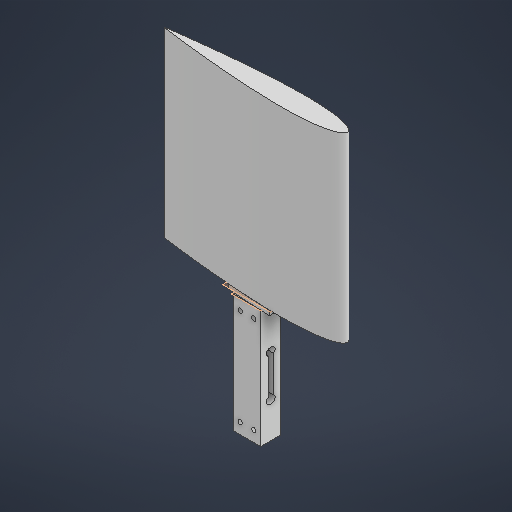
# Autodesk Inventor part: Suporte
Saved by Autodesk Inventor 2027.1 (Build 311270010, 270A)
## iProperties
Created: 2026-08-03
Part Number: Suporte
Material: Genérico
Document SubType Name: Modeling
Designer: mateu
Density: 1 g/cm^3
Appearance: Padrão
Author: mateu
Autodesk Inventor part; units mm, degrees
ref_plane "YZ Plane" through (0, 0, 0) normal (1, 0, 0) x (0, 1, 0)
ref_plane "XZ Plane" through (0, 0, 0) normal (0, 1, 0) x (-1, 0, 0)
ref_plane "XY Plane" through (0, 0, 0) normal (0, 0, 1) x (1, 0, 0)
sketch "Esboço1" plane through (0, 0, 0) normal (0, 0, 1) x (1, 0, 0)
  line L0 (-15, 65) -> (15, 65)
  line L1 (15, 65) -> (15, -65)
  line L2 (15, -65) -> (-15, -65)
  line L3 (-15, -65) -> (-15, 65)
  point P0 (0, 0)
  point P1 (0, 65)
  dimension "d0" = 130
  dimension "d1" = 65
  dimension "d2" = 30
  dimension "d3" = 0
  constraints: 8 end point, 2 parallel, 1 horizontal, 1 midpoint, 1 perpendicular
  measures "d0" distance of L1.end L0.end
  measures "d1" distance from line of point (0, 0) L0
  measures "d2" distance of L0.end L0.start
  measures "d3" horizontal distance of point (0, 65) point (0, 0)
extrude "Extrusão1" add sketch "Esboço1" along normal blind 22
sketch "Esboço2" plane through (0, 0, 0) normal (0, 0, -1) x (-1, 0, 0)
  line L0 (15, -65) -> (-15, -65) projected
  line L1 (15, 65) -> (15, -65) projected
  point P0 (0, 0)
  point P1 (7.5, -53)
  point P2 (0, -65)
  dimension "d24" = 7.5
  dimension "d25" = 12
  constraints: 1 midpoint
  measures "d24" distance from line of L1 point (7.5, -53)
  measures "d25" distance from line of L0 point (7.5, -53)
hole "Furo1" at (-7.5, -53, 0) direction (0, 0, 1) diameter 4.917 end through all thread size "M6x1" class "6H" standard "ISO Metric profile"
sketch "Esboço3" plane through (0, 0, 0) normal (0, 0, -1) x (-1, 0, 0)
  line L0 (15, -65) -> (-15, -65) projected
  circle A0 centre (7.5, -53) radius 2.4585 projected
  point P0 (0, 0)
  point P1 (-7.5, -53)
  dimension "d22" = 12
  dimension "d26" = 15
  measures "d22" distance from line of L0 point (-7.5, -53)
  measures "d26" distance of point (-7.5, -53) A0.centre
hole "Furo2" at (7.5, -53, 0) direction (0, 0, 1) diameter 4.917 end through all thread size "M6x1" class "6H" standard "ISO Metric profile"
sketch "Esboço4" plane through (0, 0, 22) normal (0, 0, 1) x (1, 0, 0)
  line L0 (15, 65) -> (-15, 65) projected
  line L1 (15, -65) -> (15, 65) projected
  point P0 (0, 0)
  point P1 (-7.5, 53)
  point P2 (7.5, 53)
  dimension "d34" = 15
  dimension "d35" = 12
  dimension "d36" = 12
  dimension "d37" = 7.5
  measures "d34" distance of point (7.5, 53) point (-7.5, 53)
  measures "d35" distance from line of L0 point (-7.5, 53)
  measures "d36" distance from line of L0 point (7.5, 53)
  measures "d37" distance from line of L1 point (7.5, 53)
hole "Furo3" at (-7.5, 53, 22) at (7.5, 53, 22) direction (0, 0, -1) diameter 4.917 end through all thread size "M6x1" class "6H" standard "ISO Metric profile"
sketch "Esboço5" plane through (-15, -65, 0) normal (-1, 0, 0) x (0, 0, 1)
  line L0 (8, 42.2) -> (8, 81.8)
  line L1 (22, 0) -> (22, 130) projected
  line L2 (13.2941, 42.5541) -> (13.2941, 81.4459)
  line L3 (0, 130) -> (0, 0) projected
  ellipse E0 centre (11, 39) end of major axis (6, 39) minor radius 4 (8, 42.2) -> (13.2941, 42.5541) ccw
  ellipse E1 centre (11, 85) end of major axis (6, 85) minor radius 4 (13.2941, 81.4459) -> (8, 81.8) ccw
  point P0 (0, 65)
  point P1 (0, 65)
  point P2 (8, 62)
  dimension "d40" = 8
  constraints: 4 end point, 2 midpoint, 1 vertical, 8 other
  measures "d40" horizontal distance of point (0, 65) point (8, 62)
extrude "Extrusão2" cut sketch "Esboço5" against normal blind 30
sketch "Esboço6" plane through (-15, 65, 0) normal (0, 1, 0) x (1, 0, 0)
  line L0 (30, 0) -> (0, 0) projected
  line L1 (30, 0) -> (30, -22) projected
  point P0 (15, 0)
  point P1 (15, -11)
  point P2 (15, 0)
  dimension "d50" = 11
  dimension "d51" = 15
  constraints: 1 midpoint
  measures "d50" distance of point (15, 0) point (15, -11)
  measures "d51" distance from line of L1 point (15, -11)
hole "Furo4" at (0, 65, 11) direction (0, -1, 0) diameter 4.917 end through all thread size "M6x1" class "6H" standard "ISO Metric profile"
ref_plane "Plano de trabalho1" through (-15, 65, 11) normal (0, 1, 0) x (1, 0, 0)
sketch "Esboço7" plane through (-15, 65, 0) normal (0, 1, 0) x (1, 0, 0)
  spline S0 degree 4 poles (-85.9155, -11.2779) (-85.8439, -11.2878) (-85.4953, -11.3359) (-84.9101, -11.4167) (-83.9238, -11.5521) (-82.8882, -11.6927) (-81.6192, -11.8648) (-80.129, -12.0648) (-78.4169, -12.2921) (-76.4894, -12.5454) (-74.3498, -12.823) (-72.0038, -13.1236) (-69.4563, -13.4446) (-66.7141, -13.7854) (-63.7826, -14.1434) (-60.6694, -14.5168) (-57.3818, -14.904) (-53.9268, -15.3029) (-50.3132, -15.7109) (-46.549, -16.1274) (-42.6432, -16.5489) (-38.605, -16.9747) (-34.4437, -17.4012) (-30.1687, -17.8282) (-25.7912, -18.2519) (-21.3189, -18.671) (-16.7725, -19.0832) (-12.1287, -19.4848) (-7.4947, -19.8798) (-2.7032, -20.2527) (2.0551, -20.6151) (6.8684, -20.956) (11.6887, -21.2762) (16.5168, -21.572) (21.3384, -21.8407) (26.1391, -22.0803) (30.9224, -22.2877) (35.6373, -22.462) (40.3236, -22.599) (44.9725, -22.6969) (49.5196, -22.7548) (53.9946, -22.7699) (58.3721, -22.741) (62.6467, -22.6675) (66.8074, -22.5469) (70.8451, -22.3803) (74.7504, -22.1661) (78.514, -21.9053) (82.1273, -21.5976) (85.5816, -21.2439) (88.8692, -20.8453) (91.9823, -20.4037) (94.9136, -19.9196) (97.6566, -19.3956) (100.2049, -18.8338) (102.5526, -18.2359) (104.6947, -17.6047) (106.6265, -16.9423) (108.3443, -16.2508) (109.8449, -15.5323) (111.1261, -14.7877) (112.1867, -14.0178) (113.0249, -13.2201) (113.6369, -12.3914) (114.0114, -11.531) (114.1354, -10.6418) (114.008, -9.7531) (113.6302, -8.8941) (113.015, -8.0678) (112.1737, -7.2733) (111.1102, -6.5075) (109.8262, -5.7678) (108.3229, -5.0551) (106.6024, -4.3702) (104.6681, -3.7152) (102.5235, -3.0923) (100.1736, -2.5034) (97.6231, -1.9513) (94.8781, -1.4379) (91.945, -0.965) (88.8302, -0.5354) (85.5411, -0.1494) (82.0855, 0.1911) (78.471, 0.4848) (74.7065, 0.7312) (70.8004, 0.9304) (66.7621, 1.0815) (62.6007, 1.1861) (58.3266, 1.2432) (53.9484, 1.2553) (49.4819, 1.223) (44.9219, 1.1481) (40.3202, 1.0315) (35.6328, 0.8761) (30.8735, 0.6853) (26.1044, 0.4588) (21.296, 0.2008) (16.4759, -0.0866) (11.6491, -0.4009) (6.8288, -0.7393) (2.0251, -1.0991) (-2.7506, -1.4782) (-7.4865, -1.8734) (-12.1725, -2.2823) (-16.7969, -2.7033) (-21.3494, -3.1325) (-25.8188, -3.5691) (-30.1955, -4.0095) (-34.4685, -4.453) (-38.6282, -4.8954) (-42.6647, -5.3367) (-46.5689, -5.7732) (-50.3314, -6.2041) (-53.9435, -6.626) (-57.3969, -7.0382) (-60.683, -7.438) (-63.7948, -7.8234) (-66.7248, -8.1926) (-69.4657, -8.544) (-72.0119, -8.8747) (-74.3568, -9.1844) (-76.4953, -9.4701) (-78.4218, -9.7309) (-80.133, -9.9648) (-81.6225, -10.1704) (-82.8907, -10.3474) (-83.9258, -10.492) (-84.9116, -10.6312) (-85.4965, -10.7142) (-85.8449, -10.7636) (-85.9164, -10.7739) knots 0 0 0 0 0 0.0063 0.010007 0.01432 0.019151 0.024442 0.030148 0.036235 0.042672 0.049434 0.056497 0.063841 0.071448 0.079299 0.087378 0.09567 0.104159 0.112831 0.121672 0.130669 0.139808 0.149077 0.158464 0.167955 0.177539 0.187194 0.196927 0.206717 0.216551 0.226428 0.236317 0.246216 0.256114 0.265998 0.275852 0.28567 0.295446 0.305162 0.314814 0.324383 0.333852 0.343216 0.352462 0.361579 0.370555 0.379378 0.388035 0.396515 0.404804 0.412889 0.420757 0.428395 0.435788 0.442923 0.449784 0.456357 0.462627 0.468581 0.47421 0.479508 0.484483 0.489162 0.493602 0.497886 0.502114 0.506398 0.510839 0.515517 0.520492 0.52579 0.531419 0.537373 0.543644 0.550217 0.557078 0.564212 0.571605 0.579243 0.587112 0.595197 0.603486 0.611965 0.620622 0.629445 0.638421 0.647538 0.656784 0.666148 0.675617 0.685175 0.694814 0.704531 0.714306 0.724136 0.734001 0.743886 0.753783 0.763683 0.773572 0.78344 0.793274 0.803064 0.812797 0.822461 0.832045 0.841536 0.850923 0.860192 0.869331 0.878328 0.887169 0.895841 0.90433 0.912622 0.920701 0.928552 0.936159 0.943503 0.950566 0.957328 0.963765 0.969852 0.975558 0.980849 0.98568 0.989993 0.9937 1 1 1 1 1
  line L0 (-85.4498, -10.7076) -> (-85.9164, -10.7739)
  line L1 (-85.7986, -11.294) -> (-87.8652, -11.0296)
  line L2 (-87.8652, -11.0296) -> (-85.7997, -10.7572)
  arc A0 (-13.9447, 8.0586) -> (-13.9447, 8.0586) centre (-12.476, -36.7013) ccw
  line L3 (96.9543, 74.8341) -> (75.7631, 39.7352)
  circle A1 centre (85.6496, 3.5164) radius 2.75
  line L4 (85.6496, 3.5164) -> (84.9837, -0.1033)
  line L5 (30, -22) -> (0, -22) projected
  line L6 (40.3546, 1.025) -> (40.3546, -22.5918)
  line L7 (-7.5118, -1.8793) -> (-7.5118, -19.8713)
  circle A2 centre (15, -11) radius 2.4585
  point P0 (15, 0)
  point P1 (-12.476, -36.7013)
  point P2 (-85.4485, -11.3424)
  point P3 (-84.8658, -11.4227)
  point P4 (-84.052, -11.5343)
  point P5 (-83.0089, -11.6763)
  point P6 (-81.739, -11.8483)
  point P7 (-80.2452, -12.0488)
  point P8 (-78.5309, -12.2765)
  point P9 (-76.6004, -12.5302)
  point P10 (-74.4581, -12.8083)
  point P11 (-72.1089, -13.1092)
  point P12 (-69.5583, -13.4309)
  point P13 (-66.8124, -13.772)
  point P14 (-63.8773, -14.1306)
  point P15 (-60.7602, -14.5046)
  point P16 (-57.4685, -14.8923)
  point P17 (-54.0093, -15.2916)
  point P18 (-50.3911, -15.7005)
  point P19 (-46.6223, -16.1172)
  point P20 (-42.7117, -16.5395)
  point P21 (-38.6685, -16.9656)
  point P22 (-34.502, -17.393)
  point P23 (-30.222, -17.8202)
  point P24 (-25.8384, -18.2445)
  point P25 (-21.3618, -18.6641)
  point P26 (-16.8022, -19.0766)
  point P27 (-12.1704, -19.4799)
  point P28 (-2.7339, -20.2486)
  point P29 (2.049, -20.6094)
  point P30 (6.8599, -20.951)
  point P31 (11.6875, -21.2709)
  point P32 (16.5209, -21.5666)
  point P33 (21.3484, -21.8354)
  point P34 (26.1591, -22.0747)
  point P35 (30.9415, -22.2821)
  point P36 (35.6622, -22.4553)
  point P37 (45.0083, -22.6895)
  point P38 (49.5672, -22.7464)
  point P39 (54.0432, -22.7606)
  point P40 (58.426, -22.7308)
  point P41 (62.7051, -22.6558)
  point P42 (66.8704, -22.5342)
  point P43 (70.9125, -22.3658)
  point P44 (74.8219, -22.1501)
  point P45 (78.5894, -21.8873)
  point P46 (82.2062, -21.5775)
  point P47 (85.6637, -21.2215)
  point P48 (88.9542, -20.8204)
  point P49 (92.0697, -20.3756)
  point P50 (95.003, -19.8883)
  point P51 (97.7474, -19.3607)
  point P52 (100.2963, -18.7946)
  point P53 (102.6438, -18.1921)
  point P54 (104.7843, -17.5556)
  point P55 (106.7131, -16.8873)
  point P56 (108.4255, -16.1894)
  point P57 (109.9175, -15.4641)
  point P58 (111.1857, -14.7135)
  point P59 (112.227, -13.9397)
  point P60 (113.0391, -13.1441)
  point P61 (113.6201, -12.3286)
  point P62 (113.9685, -11.4941)
  point P63 (114.0837, -10.6419)
  point P64 (113.9653, -9.7901)
  point P65 (113.6137, -8.957)
  point P66 (113.0295, -8.1437)
  point P67 (112.2144, -7.3513)
  point P68 (111.1701, -6.5815)
  point P69 (109.8991, -5.8357)
  point P70 (108.4043, -5.1162)
  point P71 (106.6891, -4.4249)
  point P72 (104.7579, -3.764)
  point P73 (102.6149, -3.1357)
  point P74 (100.2651, -2.5422)
  point P75 (97.714, -1.9859)
  point P76 (94.9676, -1.4688)
  point P77 (92.0325, -0.9928)
  point P78 (88.9153, -0.56)
  point P79 (85.6233, -0.1715)
  point P80 (82.1645, 0.1712)
  point P81 (78.5465, 0.4671)
  point P82 (74.778, 0.7155)
  point P83 (70.8678, 0.9162)
  point P84 (66.8251, 1.069)
  point P85 (62.6593, 1.1746)
  point P86 (58.38, 1.2332)
  point P87 (53.9972, 1.2462)
  point P88 (49.5212, 1.2148)
  point P89 (44.9625, 1.1404)
  point P90 (35.6622, 0.8703)
  point P91 (30.8974, 0.679)
  point P92 (26.1158, 0.4532)
  point P93 (21.3061, 0.1954)
  point P94 (16.4797, -0.0919)
  point P95 (11.6474, -0.4061)
  point P96 (6.8211, -0.7446)
  point P97 (2.0116, -1.1046)
  point P98 (-2.7699, -1.4838)
  point P99 (-12.2034, -2.2887)
  point P100 (-16.8336, -2.7098)
  point P101 (-21.3916, -3.1398)
  point P102 (-25.8665, -3.5766)
  point P103 (-30.2485, -4.0178)
  point P104 (-34.5269, -4.4614)
  point P105 (-38.6916, -4.9048)
  point P106 (-42.7332, -5.3464)
  point P107 (-46.6421, -5.7837)
  point P108 (-50.4093, -6.2149)
  point P109 (-54.0259, -6.6376)
  point P110 (-57.4835, -7.0503)
  point P111 (-60.7738, -7.4506)
  point P112 (-63.8894, -7.8366)
  point P113 (-66.8231, -8.2064)
  point P114 (-69.5676, -8.5581)
  point P115 (-72.117, -8.8896)
  point P116 (-74.465, -9.1995)
  point P117 (-76.6063, -9.4858)
  point P118 (-78.5358, -9.7469)
  point P119 (-80.2491, -9.9812)
  point P120 (-81.7421, -10.1875)
  point P121 (-83.0114, -10.3643)
  point P122 (-84.0539, -10.5103)
  point P123 (-84.8673, -10.6251)
  constraints: 14 end point, 3 centre point, 2 point on circle, 1 parallel, 1 vertical, 132 other
extrude "Extrusão3" add sketch "Esboço7" along normal blind 5 contours L7 S0 A0 L5 | L5 A0 S0 | S0 L6 A0
sketch "Esboço8" plane through (-15, 65, 0) normal (0, -1, 0) x (1, 0, 0)
  point P0 (15, 0)
  point P1 (36.2049, 3.5099)
  point P2 (35.8652, 17.7373)
  point P3 (-4.184, 5.5484)
  point P4 (-4.184, 16.3783)
hole "Furo5" at (21.2049, 65, 3.5099) at (20.8652, 65, 17.7373) at (-19.184, 65, 5.5484) at (-19.184, 65, 16.3783) direction (0, 1, 0) diameter 4.917 end through all thread size "M6x1" class "6H" standard "ISO Metric profile"
ref_plane "Plano de trabalho2" through (-22.5118, 70, 10.8753) normal (0, 1, 0) x (0.9999982, 0, -0.0019192)
sketch "Esboço9" plane through (-22.5118, 70, 10.8753) normal (0, 1, 0) x (0.9999982, 0, -0.0019192)
  spline S0 degree 4 poles (-78.9155, -0.2779) (-78.8439, -0.2878) (-78.4953, -0.3359) (-77.9101, -0.4167) (-76.9238, -0.5521) (-75.8882, -0.6927) (-74.6192, -0.8648) (-73.129, -1.0648) (-71.4169, -1.2921) (-69.4894, -1.5454) (-67.3498, -1.823) (-65.0038, -2.1236) (-62.4563, -2.4446) (-59.7141, -2.7854) (-56.7826, -3.1434) (-53.6694, -3.5168) (-50.3818, -3.904) (-46.9268, -4.3029) (-43.3132, -4.7109) (-39.549, -5.1274) (-35.6432, -5.5489) (-31.605, -5.9747) (-27.4437, -6.4012) (-23.1687, -6.8282) (-18.7912, -7.2519) (-14.3189, -7.671) (-9.7725, -8.0832) (-5.1287, -8.4848) (-0.4947, -8.8798) (4.2968, -9.2527) (9.0551, -9.6151) (13.8684, -9.956) (18.6887, -10.2762) (23.5168, -10.572) (28.3384, -10.8407) (33.1391, -11.0803) (37.9224, -11.2877) (42.6373, -11.462) (47.3236, -11.599) (51.9725, -11.6969) (56.5196, -11.7548) (60.9946, -11.7699) (65.3721, -11.741) (69.6467, -11.6675) (73.8074, -11.5469) (77.8451, -11.3803) (81.7504, -11.1661) (85.514, -10.9053) (89.1273, -10.5976) (92.5816, -10.2439) (95.8692, -9.8453) (98.9823, -9.4037) (101.9136, -8.9196) (104.6566, -8.3956) (107.2049, -7.8338) (109.5526, -7.2359) (111.6947, -6.6047) (113.6265, -5.9423) (115.3443, -5.2508) (116.8449, -4.5323) (118.1261, -3.7877) (119.1867, -3.0178) (120.0249, -2.2201) (120.6369, -1.3914) (121.0114, -0.531) (121.1354, 0.3582) (121.008, 1.2469) (120.6302, 2.1059) (120.015, 2.9322) (119.1737, 3.7267) (118.1102, 4.4925) (116.8262, 5.2322) (115.3229, 5.9449) (113.6024, 6.6298) (111.6681, 7.2848) (109.5235, 7.9077) (107.1736, 8.4966) (104.6231, 9.0487) (101.8781, 9.5621) (98.945, 10.035) (95.8302, 10.4646) (92.5411, 10.8506) (89.0855, 11.1911) (85.471, 11.4848) (81.7065, 11.7312) (77.8004, 11.9304) (73.7621, 12.0815) (69.6007, 12.1861) (65.3266, 12.2432) (60.9484, 12.2553) (56.4819, 12.223) (51.9219, 12.1481) (47.3202, 12.0315) (42.6328, 11.8761) (37.8735, 11.6853) (33.1044, 11.4588) (28.296, 11.2008) (23.4759, 10.9134) (18.6491, 10.5991) (13.8288, 10.2607) (9.0251, 9.9009) (4.2494, 9.5218) (-0.4865, 9.1266) (-5.1725, 8.7177) (-9.7969, 8.2967) (-14.3494, 7.8675) (-18.8188, 7.4309) (-23.1955, 6.9905) (-27.4685, 6.547) (-31.6282, 6.1046) (-35.6647, 5.6633) (-39.5689, 5.2268) (-43.3314, 4.7959) (-46.9435, 4.374) (-50.3969, 3.9618) (-53.683, 3.562) (-56.7948, 3.1766) (-59.7248, 2.8074) (-62.4657, 2.456) (-65.0119, 2.1253) (-67.3568, 1.8156) (-69.4953, 1.5299) (-71.4218, 1.2691) (-73.133, 1.0352) (-74.6225, 0.8296) (-75.8907, 0.6526) (-76.9258, 0.508) (-77.9116, 0.3688) (-78.4965, 0.2858) (-78.8449, 0.2364) (-78.9164, 0.2261) knots 0 0 0 0 0 0.0063 0.010007 0.01432 0.019151 0.024442 0.030148 0.036235 0.042672 0.049434 0.056497 0.063841 0.071448 0.079299 0.087378 0.09567 0.104159 0.112831 0.121672 0.130669 0.139808 0.149077 0.158464 0.167955 0.177539 0.187194 0.196927 0.206717 0.216551 0.226428 0.236317 0.246216 0.256114 0.265998 0.275852 0.28567 0.295446 0.305162 0.314814 0.324383 0.333852 0.343216 0.352462 0.361579 0.370555 0.379378 0.388035 0.396515 0.404804 0.412889 0.420757 0.428395 0.435788 0.442923 0.449784 0.456357 0.462627 0.468581 0.47421 0.479508 0.484483 0.489162 0.493602 0.497886 0.502114 0.506398 0.510839 0.515517 0.520492 0.52579 0.531419 0.537373 0.543644 0.550217 0.557078 0.564212 0.571605 0.579243 0.587112 0.595197 0.603486 0.611965 0.620622 0.629445 0.638421 0.647538 0.656784 0.666148 0.675617 0.685175 0.694814 0.704531 0.714306 0.724136 0.734001 0.743886 0.753783 0.763683 0.773572 0.78344 0.793274 0.803064 0.812797 0.822461 0.832045 0.841536 0.850923 0.860192 0.869331 0.878328 0.887169 0.895841 0.90433 0.912622 0.920701 0.928552 0.936159 0.943503 0.950566 0.957328 0.963765 0.969852 0.975558 0.980849 0.98568 0.989993 0.9937 1 1 1 1 1
  line L0 (-78.4498, 0.2924) -> (-78.9164, 0.2261)
  line L1 (-78.7986, -0.294) -> (-76.8947, 29.1141)
  line L2 (-76.8947, 29.1141) -> (-78.7997, 0.2428)
  arc A0 (-6.9447, 19.0586) -> (-6.9447, 19.0586) centre (-5.476, -25.7013) ccw
  circle A1 centre (92.6496, 14.5164) radius 2.75
  line L3 (92.6496, 14.5164) -> (94.5601, -9.9983)
  line L4 (37, -11) -> (7, -11)
  circle A2 centre (22, 0) radius 2.4585
  point P0 (22.5326, 10.8321)
  point P1 (22, 11)
  point P2 (-100.5055, 47.4424)
  point P3 (-78.4485, -0.3424)
  point P4 (-77.8658, -0.4227)
  point P5 (-77.052, -0.5343)
  point P6 (-76.0089, -0.6763)
  point P7 (-74.739, -0.8483)
  point P8 (-73.2452, -1.0488)
  point P9 (-71.5309, -1.2765)
  point P10 (-69.6004, -1.5302)
  point P11 (-67.4581, -1.8083)
  point P12 (-65.1089, -2.1092)
  point P13 (-62.5583, -2.4309)
  point P14 (-59.8124, -2.772)
  point P15 (-56.8773, -3.1306)
  point P16 (-53.7602, -3.5046)
  point P17 (-50.4685, -3.8923)
  point P18 (-47.0093, -4.2916)
  point P19 (-43.3911, -4.7005)
  point P20 (-39.6223, -5.1172)
  point P21 (-35.7117, -5.5395)
  point P22 (-31.6685, -5.9656)
  point P23 (-27.502, -6.393)
  point P24 (-23.222, -6.8202)
  point P25 (-18.8384, -7.2445)
  point P26 (-14.3618, -7.6641)
  point P27 (-9.8022, -8.0766)
  point P28 (-5.1704, -8.4799)
  point P29 (-0.5118, -8.8713)
  point P30 (4.2661, -9.2486)
  point P31 (9.049, -9.6094)
  point P32 (13.8599, -9.951)
  point P33 (18.6875, -10.2709)
  point P34 (23.5209, -10.5666)
  point P35 (28.3484, -10.8354)
  point P36 (33.1591, -11.0747)
  point P37 (37.9415, -11.2821)
  point P38 (42.6622, -11.4553)
  point P39 (47.3546, -11.5918)
  point P40 (52.0083, -11.6895)
  point P41 (56.5672, -11.7464)
  point P42 (61.0432, -11.7606)
  point P43 (65.426, -11.7308)
  point P44 (69.7051, -11.6558)
  point P45 (73.8704, -11.5342)
  point P46 (77.9125, -11.3658)
  point P47 (81.8219, -11.1501)
  point P48 (85.5894, -10.8873)
  point P49 (89.2062, -10.5775)
  point P50 (92.6637, -10.2215)
  point P51 (95.9542, -9.8204)
  point P52 (99.0697, -9.3756)
  point P53 (102.003, -8.8883)
  point P54 (104.7474, -8.3607)
  point P55 (107.2963, -7.7946)
  point P56 (109.6438, -7.1921)
  point P57 (111.7843, -6.5556)
  point P58 (113.7131, -5.8873)
  point P59 (115.4255, -5.1894)
  point P60 (116.9175, -4.4641)
  point P61 (118.1857, -3.7135)
  point P62 (119.227, -2.9397)
  point P63 (120.0391, -2.1441)
  point P64 (120.6201, -1.3286)
  point P65 (120.9685, -0.4941)
  point P66 (121.0837, 0.3581)
  point P67 (120.9653, 1.2099)
  point P68 (120.6137, 2.043)
  point P69 (120.0295, 2.8563)
  point P70 (119.2144, 3.6487)
  point P71 (118.1701, 4.4185)
  point P72 (116.8991, 5.1643)
  point P73 (115.4043, 5.8838)
  point P74 (113.6891, 6.5751)
  point P75 (111.7579, 7.236)
  point P76 (109.6149, 7.8643)
  point P77 (107.2651, 8.4578)
  point P78 (104.714, 9.0141)
  point P79 (101.9676, 9.5312)
  point P80 (99.0325, 10.0072)
  point P81 (95.9153, 10.44)
  point P82 (92.6233, 10.8285)
  point P83 (89.1645, 11.1712)
  point P84 (85.5465, 11.4671)
  point P85 (81.778, 11.7155)
  point P86 (77.8678, 11.9162)
  point P87 (73.8251, 12.069)
  point P88 (69.6593, 12.1746)
  point P89 (65.38, 12.2332)
  point P90 (60.9972, 12.2462)
  point P91 (56.5212, 12.2148)
  point P92 (51.9625, 12.1404)
  point P93 (47.3546, 12.025)
  point P94 (42.6622, 11.8703)
  point P95 (37.8974, 11.679)
  point P96 (33.1158, 11.4532)
  point P97 (28.3061, 11.1954)
  point P98 (23.4797, 10.9081)
  point P99 (18.6474, 10.5939)
  point P100 (13.8211, 10.2554)
  point P101 (9.0116, 9.8954)
  point P102 (4.2301, 9.5162)
  point P103 (-0.5118, 9.1207)
  point P104 (-5.2034, 8.7113)
  point P105 (-9.8336, 8.2902)
  point P106 (-14.3916, 7.8602)
  point P107 (-18.8665, 7.4234)
  point P108 (-23.2485, 6.9822)
  point P109 (-27.5269, 6.5386)
  point P110 (-31.6916, 6.0952)
  point P111 (-35.7332, 5.6536)
  point P112 (-39.6421, 5.2163)
  point P113 (-43.4093, 4.7851)
  point P114 (-47.0259, 4.3624)
  point P115 (-50.4835, 3.9497)
  point P116 (-53.7738, 3.5494)
  point P117 (-56.8894, 3.1634)
  point P118 (-59.8231, 2.7936)
  point P119 (-62.5676, 2.4419)
  point P120 (-65.117, 2.1104)
  point P121 (-67.465, 1.8005)
  point P122 (-69.6063, 1.5142)
  point P123 (-71.5358, 1.2531)
  point P124 (-73.2491, 1.0188)
  point P125 (-74.7421, 0.8125)
  point P126 (-76.0114, 0.6357)
  point P127 (-77.0539, 0.4897)
  point P128 (-77.8673, 0.3749)
  point P129 (-78.7635, 0.2479)
  constraints: 10 end point, 3 centre point, 2 point on circle, 132 other
extrude "Extrusão4" add sketch "Esboço9" along normal blind 200 contours L1 S0 A0 | A0 S0 L4 | L4 A0 S0 | A0 S0 L3 | L3 S0 | A2
